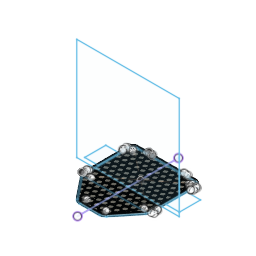
621 Chassis (Autodesk Fusion 360 design; units mm, degrees)
part number: 2026-02-18-00-04-41-213
Autodesk Fusion 360 part; units mm, degrees
note: some values were not read from the file. Set by a fixed rule: which sketch regions a step uses.
(part 1 of 3)
sketch "Sketch1" plane through (0, 0, 0) normal (0, 0, 1) x (1, 0, 0)
  line L0 (101.6, -101.6) -> (-101.6, -101.6)
  line L1 (-101.6, -101.6) -> (-101.6, 101.6)
  line L2 (-101.6, 101.6) -> (101.6, 101.6)
  line L3 (101.6, 101.6) -> (101.6, -101.6)
  line L4 (101.6, -101.6) -> (-101.6, 101.6) construction
  line L5 (-101.6, -101.6) -> (101.6, 101.6) construction
  dimension "d1" = 203.2
  dimension "d2" = 203.2
  constraint horizontal L0
  constraint perpendicular L0 L1
  constraint parallel L0 L2
  constraint parallel L1 L3
  constraint coincident L4 origin
  constraint coincident L5 origin
  measures "d1" distance of L1.end L2.end
  measures "d2" distance of L0.end L1.end
sketch "Sketch2" plane through (0, 0, 0) normal (0, 0, 1) x (1, 0, 0)
sketch "Sketch3" plane through (0, 0, 0) normal (0, 0, 1) x (1, 0, 0)
  line L0 (101.6, 101.6) -> (-101.6, 101.6)
  line L1 (-101.6, 101.6) -> (-101.6, -101.6)
  line L2 (-101.6, -101.6) -> (101.6, -101.6)
  line L3 (101.6, -101.6) -> (101.6, 101.6)
  line L4 (101.6, 101.6) -> (-101.6, -101.6) construction
  line L5 (-101.6, 101.6) -> (101.6, -101.6) construction
  dimension "d5" = 203.2
  dimension "d6" = 203.2
  constraint horizontal L0
  constraint perpendicular L0 L1
  constraint parallel L0 L2
  constraint parallel L1 L3
  constraint coincident L4 origin
  constraint coincident L5 origin
  measures "d5" distance of L1.end L2.end
  measures "d6" distance of L0.end L1.end
sketch "Sketch4" plane through (0, 0, 0) normal (0, 1, 0) x (1, 0, 0)
  line L0 (-101.6, 0) -> (101.6, 0)
  line L1 (101.6, 0) -> (101.6, -203.2)
  line L2 (101.6, -203.2) -> (-101.6, -203.2)
  line L3 (-101.6, -203.2) -> (-101.6, 0)
  dimension "d7" = 203.2
  dimension "d8" = 203.2
  constraint horizontal L0
  constraint vertical L1
  constraint horizontal L2
  constraint vertical L3
  measures "d7" distance of L0.start L0.end
  measures "d8" distance of L0.start L2.end
sketch "Sketch5" plane through (0, 0, 0) normal (0, 0, 1) x (1, 0, 0)
  line L0 (55, 75) -> (-55, 75)
  line L1 (-65, 65) -> (-65, -20.4398)
  line L2 (-65, -25) -> (65, -25)
  line L3 (65, -20.4398) -> (65, 65)
  line L4 (65, 75) -> (-65, -25) construction
  line L5 (-65, 75) -> (65, -25) construction
  line L6 (-62.1513, -28.5609) -> (-28.9032, -70.121)
  line L7 (-18.7519, -75) -> (18.7519, -75)
  line L8 (28.9032, -70.121) -> (62.1513, -28.5609)
  line L9 (67, -21.1414) -> (67, 69)
  line L10 (59, 77) -> (41, 77)
  line L11 (-67, 69) -> (-67, -9)
  line L12 (-64.1513, -29.2624) -> (-29.8644, -72.121)
  line L13 (-19.7131, -77) -> (19.7131, -77)
  line L14 (29.8644, -72.121) -> (64.1513, -29.2624)
  line L15 (-59, 77) -> (-41, 77)
  line L16 (0, 100) -> (0, -100)
  line L17 (-40, 77) -> (29, 77)
  line L18 (-30, 78) -> (-30, 81)
  line L19 (-31, 82) -> (-39, 82)
  line L20 (-40, 81) -> (-40, 78)
  line L21 (31, 82) -> (39, 82)
  line L22 (30, 78) -> (30, 81)
  line L23 (40, 81) -> (40, 78)
  arc A0 (-39, 82) -> (-40, 81) centre (-39, 81) ccw
  arc A1 (-30, 81) -> (-31, 82) centre (-31, 81) ccw
  arc A2 (-30, 78) -> (-29, 77) centre (-29, 78) ccw
  arc A3 (-41, 77) -> (-40, 78) centre (-41, 78) ccw
  arc A4 (40, 78) -> (41, 77) centre (41, 78) ccw
  arc A5 (29, 77) -> (30, 78) centre (29, 78) ccw
  line L24 (29, 77) -> (51.3644, 77)
  line L25 (-41, 77) -> (-29, 77)
  arc A6 (31, 82) -> (30, 81) centre (31, 81) ccw
  arc A7 (40, 81) -> (39, 82) centre (39, 81) ccw
  circle A8 centre (-37.5, 79.5) radius 1.5
  circle A9 centre (-32.5, 79.5) radius 1.5
  circle A10 centre (37.5, 79.5) radius 1.5
  circle A11 centre (32.5, 79.5) radius 1.5
  arc A12 (-55, 75) -> (-65, 65) centre (-55, 65) ccw
  arc A13 (-59, 77) -> (-67, 69) centre (-59, 69) ccw
  arc A14 (65, 65) -> (55, 75) centre (55, 65) ccw
  arc A15 (67, 69) -> (59, 77) centre (59, 69) ccw
  arc A16 (-29.8644, -72.121) -> (-19.7131, -77) centre (-19.7131, -64) ccw
  arc A17 (19.7131, -77) -> (29.8644, -72.121) centre (19.7131, -64) ccw
  arc A18 (18.7519, -75) -> (28.9032, -70.121) centre (18.7519, -62) ccw
  arc A19 (-28.9032, -70.121) -> (-18.7519, -75) centre (-18.7519, -62) ccw
  arc A20 (-67, -21.1414) -> (-64.1513, -29.2624) centre (-54, -21.1414) ccw
  arc A21 (-65, -20.4398) -> (-62.1513, -28.5609) centre (-52, -20.4398) ccw
  arc A22 (62.1513, -28.5609) -> (65, -20.4398) centre (52, -20.4398) ccw
  arc A23 (64.1513, -29.2624) -> (67, -21.1414) centre (54, -21.1414) ccw
  line L26 (-67.9937, -20) -> (-71, -20)
  line L27 (-72, -19) -> (-72, -11)
  line L28 (-71, -10) -> (-68, -10)
  line L29 (-67, -10) -> (-67, -20)
  circle A24 centre (-69.5, -17.5) radius 1.5
  circle A25 centre (-69.5, -12.5) radius 1.5
  arc A26 (-71, -10) -> (-72, -11) centre (-71, -11) ccw
  arc A27 (-72, -19) -> (-71, -20) centre (-71, -19) ccw
  line L30 (-66.9937, -20.9996) -> (-66.9935, -21.5528)
  arc A28 (-68, -10) -> (-67, -9) centre (-68, -9) ccw
  arc A29 (-66.9937, -20.9996) -> (-67.9937, -20) centre (-67.9937, -21) ccw
  arc A30 (72, -11) -> (71, -10) centre (71, -11) ccw
  arc A31 (71, -20) -> (72, -19) centre (71, -19) ccw
  circle A32 centre (69.5, -17.5) radius 1.5
  line L31 (67.9937, -20) -> (71, -20)
  line L32 (71, -10) -> (68, -10)
  line L33 (72, -19) -> (72, -11)
  circle A33 centre (69.5, -12.5) radius 1.5
  arc A34 (67, -9) -> (68, -10) centre (68, -9) ccw
  arc A35 (67.9937, -20) -> (66.9937, -20.9996) centre (67.9937, -21) ccw
  line L34 (-67, -9) -> (-67, -20.888)
  circle A36 centre (-69.5, -12.5) radius 1.5
  arc A37 (-72, -19) -> (-71, -20) centre (-71, -19) ccw
  line L35 (-71, -10) -> (-68, -10)
  line L36 (-72, -19) -> (-72, -11)
  circle A38 centre (-69.5, -17.5) radius 1.5
  line L37 (-67.9937, -20) -> (-71, -20)
  arc A39 (-71, -10) -> (-72, -11) centre (-71, -11) ccw
  arc A40 (-66.9937, 57.0004) -> (-67.9937, 58) centre (-67.9937, 57) ccw
  line L38 (-67.9937, 58) -> (-71, 58)
  arc A41 (-72, 59) -> (-71, 58) centre (-71, 59) ccw
  line L39 (-72, 59) -> (-72, 67)
  arc A42 (-71, 68) -> (-72, 67) centre (-71, 67) ccw
  line L40 (-71, 68) -> (-68, 68)
  arc A43 (-68, 68) -> (-67, 69) centre (-68, 69) ccw
  circle A44 centre (-69.5, 65.5) radius 1.5
  circle A45 centre (-69.5, 60.5) radius 1.5
  line L41 (-67, 68) -> (-67, 58)
  line L42 (-67, 69) -> (-67, 57.112)
  line L43 (72, 59) -> (72, 67)
  circle A46 centre (69.5, 65.5) radius 1.5
  arc A47 (67.9937, 58) -> (66.9937, 57.0004) centre (67.9937, 57) ccw
  line L44 (67, 69) -> (67, 57.112)
  line L45 (67.9937, 58) -> (71, 58)
  arc A48 (71, 58) -> (72, 59) centre (71, 59) ccw
  line L46 (71, 68) -> (68, 68)
  circle A49 centre (69.5, 60.5) radius 1.5
  arc A50 (67, 69) -> (68, 68) centre (68, 69) ccw
  line L47 (67, 68) -> (67, 58)
  arc A51 (72, 67) -> (71, 68) centre (71, 67) ccw
  point P0 (0, 25)
  point P1 (-30, 77)
  point P2 (-40, 82)
  point P3 (-72, -20)
  point P4 (72, -20)
  point P5 (-68, -9)
  point P6 (-72, -20)
  point P7 (-67.9937, -21)
  dimension "d9" = 130
  dimension "d10" = 100
  dimension "d12" = 10
  dimension "d13" = 5
  dimension "d14" = 1
  dimension "d15" = 1
  dimension "d16" = 1
  dimension "d17" = 1
  dimension "d18" = 1
  dimension "d19" = 3
  dimension "d20" = 3
  dimension "d23" = 10
  dimension "d24" = 8
  dimension "d25" = 10
  dimension "d26" = 8
  dimension "d27" = 13
  dimension "d32" = 2.5
  dimension "d33" = 2.5
  dimension "d34" = 5
  dimension "d35" = 30
  dimension "d36" = 30
  dimension "d48" = 5
  dimension "d49" = 10
  dimension "d50" = 3
  dimension "d51" = 3
  dimension "d52" = 2.5
  dimension "d53" = 5
  dimension "d54" = 2.5
  dimension "d55" = 1
  dimension "d56" = 1
  dimension "d59" = 3
  dimension "d60" = 3
  dimension "d61" = 2.5
  dimension "d62" = 5
  dimension "d63" = 2.5
  dimension "d64" = 1
  dimension "d65" = 10
  dimension "d66" = 3
  dimension "d67" = 3
  dimension "d68" = 2.5
  dimension "d69" = 5
  dimension "d70" = 2.5
  dimension "d71" = 1
  dimension "d72" = 1
  constraint horizontal L0
  constraint perpendicular L0 L1
  constraint parallel L0 L2
  constraint parallel L1 L3
  constraint coincident L4 P0
  constraint coincident L5 P0
  constraint parallel L2 L7
  constraint vertical L16
  constraint horizontal L17
  constraint vertical L18
  constraint horizontal L19
  constraint vertical L20
  constraint coincident L10 L17.start
  constraint coincident P2 L19
  constraint coincident P2 L20
  constraint tangent L19 A0
  constraint tangent L20 A0
  constraint tangent L18 A1
  constraint tangent L19 A1
  constraint equal A0 A1
  constraint coincident P1 L18
  constraint tangent L10 A2
  constraint tangent L18 A2
  constraint coincident L17.start L20
  constraint tangent L15 A3
  constraint tangent L20 A3
  constraint coincident L10 A2.end
  constraint tangent L10 A4
  constraint tangent L23 A4
  constraint coincident P1 L17
  constraint tangent L22 A5
  constraint tangent L17 A5
  constraint equal A4 A5
  constraint coincident L10 L24.end
  constraint tangent A2 L25
  constraint tangent L21 A6
  constraint tangent L22 A6
  constraint tangent L21 A7
  constraint tangent L23 A7
  constraint equal A6 A7
  constraint symmetric L16 A8 A10
  constraint symmetric L16 A9 A11
  constraint coincident L5.start L0
  constraint coincident L5.start L1
  constraint tangent L0 A12
  constraint tangent L1 A12
  constraint tangent L11 A13
  constraint tangent L15 A13
  constraint coincident L4.start L0
  constraint coincident L4.start L3
  constraint tangent L0 A14
  constraint tangent L3 A14
  constraint tangent L9 A15
  constraint tangent L10 A15
  constraint tangent L12 A16
  constraint tangent L13 A16
  constraint tangent L13 A17
  constraint tangent L14 A17
  constraint equal A16 A17
  constraint tangent L7 A18
  constraint tangent L8 A18
  constraint equal A16 A18
  constraint tangent L6 A19
  constraint tangent L7 A19
  constraint equal A16 A19
  constraint tangent L11 A20
  constraint tangent L12 A20
  constraint equal A16 A20
  constraint coincident L2.start L1
  constraint coincident L2.start L6
  constraint tangent L1 A21
  constraint tangent L6 A21
  constraint equal A16 A21
  constraint coincident L2.end L3
  constraint coincident L2.end L8
  constraint tangent L3 A22
  constraint tangent L8 A22
  constraint equal A16 A22
  constraint tangent L9 A23
  constraint tangent L14 A23
  constraint equal A16 A23
  constraint horizontal L26
  constraint vertical L27
  constraint horizontal L28
  constraint vertical L29
  constraint tangent L27 A26
  constraint tangent L28 A26
  constraint coincident P6 L26
  constraint coincident P6 L27
  constraint tangent L26 A27
  constraint tangent L27 A27
  constraint equal A26 A27
  constraint coincident A20 L30.end
  constraint coincident L11 A20.start
  constraint tangent L28 A28
  constraint tangent L11 A28
  constraint coincident L29.end L26
  constraint tangent L26 A29
  constraint tangent L30 A29
  constraint equal A28 A29
  constraint symmetric L16 P6 P4
  constraint symmetric L16 A24 A32
  constraint symmetric L16 A25 A33
  constraint symmetric L16 L27.end A30.start
  constraint symmetric L16 L28.start A30.end
  constraint symmetric L16 A26 A30
  constraint symmetric L16 L26.end A31.start
  constraint symmetric L16 L27.start A31.end
  constraint symmetric L16 A27 A31
  constraint symmetric L16 L28.end L32.end
  constraint symmetric L16 L11.end A34.start
  constraint symmetric L16 A28 A34
  constraint symmetric L16 L26.start L31.start
  constraint symmetric L16 L30.start A35.end
  constraint symmetric L16 A29 A35
  constraint coincident A29 L34.end
  constraint tangent A28 L34
  constraint horizontal L37
  constraint vertical L36
  constraint horizontal L35
  constraint tangent L36 A39
  constraint tangent L35 A39
  constraint coincident P6 L37
  constraint coincident P6 L36
  constraint tangent A37 L37
  constraint tangent A37 L36
  constraint equal A37 A39
  constraint horizontal L38
  constraint vertical L39
  constraint horizontal L40
  constraint vertical L41
  constraint tangent L39 A42
  constraint tangent A42 L40
  constraint tangent L38 A41
  constraint tangent A41 L39
  constraint equal A41 A42
  constraint tangent L40 A43
  constraint coincident L41.end L38
  constraint tangent A40 L38
  constraint equal A40 A43
  constraint coincident L42.end A40
  constraint tangent A43 L42
  constraint symmetric L16 A41.start L43.start
  constraint symmetric L16 L40.end L46.end
  constraint symmetric L16 L11.start L9.end
  constraint symmetric L16 L38.end L45.end
  constraint symmetric L16 L41.start L47.start
  constraint symmetric L16 L39.end L43.end
  constraint symmetric L16 L41.end L47.end
  constraint symmetric L16 A42.start L46.start
  constraint symmetric L16 A40.end A47.start
  constraint symmetric L16 A40.start A47.end
  constraint symmetric L16 L42.end L44.end
  constraint symmetric L16 A40 A47
  constraint symmetric L16 A41 A48
  constraint symmetric L16 A42 A51
  constraint symmetric L16 A43 A50
  constraint symmetric L16 A44 A46
  constraint symmetric L16 A45 A49
  measures "d9" distance of L2.start L2.end
  measures "d10" distance of L5.start L2.start
  measures "d12" distance of L17.start P1
  measures "d13" distance of L17.start P2
  measures "d14" radius of A0
  measures "d15" radius of A2
  measures "d16" radius of A3
  measures "d17" radius of A4
  measures "d18" radius of A6
  measures "d19" diameter of A8
  measures "d20" diameter of A9
  measures "d23" radius of A12
  measures "d24" radius of A13
  measures "d25" radius of A14
  measures "d26" radius of A15
  measures "d27" radius of A16
  measures "d32" distance of L20 A8.centre
  measures "d33" distance of L18 A9.centre
  measures "d34" distance of A8.centre A9.centre
  measures "d35" distance of L16 L22
  measures "d36" distance of L16 L18
  measures "d48" distance of L29.end P6
  measures "d49" distance of L29.end L29.start
  measures "d50" diameter of A24
  measures "d51" diameter of A25
  measures "d52" distance of L26 A24.centre
  measures "d53" distance of A24.centre A25.centre
  measures "d54" distance of L28 A25.centre
  measures "d55" radius of A26
  measures "d56" radius of A28
  measures "d59" diameter of A38
  measures "d60" diameter of A36
  measures "d61" distance of A24.centre L37
  measures "d62" distance of A25.centre A24.centre
  measures "d63" distance of A25.centre L35
  measures "d64" radius of A39
  measures "d65" distance of L41.start L41.end
  measures "d66" diameter of A45
  measures "d67" diameter of A44
  measures "d68" distance of A45.centre L38
  measures "d69" distance of A44.centre A45.centre
  measures "d70" distance of A44.centre L40
  measures "d71" radius of A42
  measures "d72" radius of A43
sketch "Wheels" plane through (0, 0, 0) normal (0, 0, 1) x (1, 0, 0)
  line L0 (-67, 50) -> (-94, 50)
  line L1 (-94, 50) -> (-94, 8)
  line L2 (-94, 8) -> (-67, 8)
  line L3 (-67, 8) -> (-67, 50)
  line L4 (0, 100) -> (0, -100)
  line L5 (94, 50) -> (94, 8)
  line L6 (67, 50) -> (94, 50)
  line L7 (94, 8) -> (67, 8)
  line L8 (67, 8) -> (67, 50)
  dimension "d21" = 27
  dimension "d22" = 42
  constraint horizontal L0
  constraint vertical L1
  constraint horizontal L2
  constraint vertical L3
  constraint symmetric L0.start L4 L6.start
  constraint symmetric L0.end L4 L5.start
  constraint symmetric L1.end L4 L5.end
  constraint symmetric L2.end L4 L7.end
  measures "d21" distance of L0.start L0.end
  measures "d22" distance of L0.start L2.end
extrude "Extrude2" add sketch "Sketch5" along normal blind 2 contours L0 L3 L7 L8 L9 L10 L13 L14 L16 L17 L24 A14 A15 A17 A18 A22 A23 L44 L47 | L0 L1 L6 L7 L11 L12 L13 L15 L16 L17 L25 A12 A13 A16 A19 A20 A21 L29 L30 A29 L34 L41 L42 makes body 1
extrude "Extrude3" add sketch "Sketch5" along normal blind 1.5 contours L17 L18 L19 L20 A0 A1 A2 A3 L25 | L21 L22 L23 A4 A5 L24 A6 A7 bodies 1
extrude "Extrude4" add 1 faces at (13.6667, 75.6667, 2) along direction (0, 0, 1) blind 2 on bodies 1 bodies 1
sketch "hex" plane through (0, 0, 0) normal (0, 0, 1) x (1, 0, 0)
  arc A0 (-55, 75) -> (-65, 65) centre (-55, 65) ccw
  line L0 (-65, 65) -> (-65, -20.4398)
  arc A1 (-65, -20.4398) -> (-62.1513, -28.5609) centre (-52, -20.4398) ccw
  line L1 (-62.1513, -28.5609) -> (-28.9032, -70.121)
  arc A2 (-28.9032, -70.121) -> (-18.7519, -75) centre (-18.7519, -62) ccw
  line L2 (-18.7519, -75) -> (18.7519, -75)
  arc A3 (18.7519, -75) -> (28.9032, -70.121) centre (18.7519, -62) ccw
  line L3 (28.9032, -70.121) -> (62.1513, -28.5609)
  arc A4 (62.1513, -28.5609) -> (65, -20.4398) centre (52, -20.4398) ccw
  line L4 (65, -20.4398) -> (65, 65)
  arc A5 (65, 65) -> (55, 75) centre (55, 65) ccw
  line L5 (55, 75) -> (-55, 75)
  line L6 (5, 2.8868) -> (0, 5.7735)
  line L7 (0, 5.7735) -> (-5, 2.8868)
  line L8 (-5, 2.8868) -> (-5, -2.8868)
  line L9 (-5, -2.8868) -> (0, -5.7735)
  line L10 (0, -5.7735) -> (5, -2.8868)
  line L11 (5, -2.8868) -> (5, 2.8868)
  line L12 (0, 0) -> (5, 0)
  line L13 (0, 0) -> (2.5, 4.3301)
  line L14 (-150, -66.9726) -> (-155, -69.8594)
  line L15 (-145, -69.8594) -> (-150, -66.9726)
  line L16 (-145, -75.6329) -> (-145, -69.8594)
  line L17 (-155, -69.8594) -> (-155, -75.6329)
  line L18 (-155, -75.6329) -> (-150, -78.5196)
  line L19 (-150, -78.5196) -> (-145, -75.6329)
  line L20 (-138, -66.9726) -> (-143, -69.8594)
  line L21 (-133, -69.8594) -> (-138, -66.9726)
  line L22 (-133, -75.6329) -> (-133, -69.8594)
  line L23 (-143, -69.8594) -> (-143, -75.6329)
  line L24 (-143, -75.6329) -> (-138, -78.5196)
  line L25 (-138, -78.5196) -> (-133, -75.6329)
  line L26 (-126, -66.9726) -> (-131, -69.8594)
  line L27 (-121, -69.8594) -> (-126, -66.9726)
  line L28 (-121, -75.6329) -> (-121, -69.8594)
  line L29 (-131, -69.8594) -> (-131, -75.6329)
  line L30 (-131, -75.6329) -> (-126, -78.5196)
  line L31 (-126, -78.5196) -> (-121, -75.6329)
  line L32 (-114, -66.9726) -> (-119, -69.8594)
  line L33 (-109, -69.8594) -> (-114, -66.9726)
  line L34 (-109, -75.6329) -> (-109, -69.8594)
  line L35 (-119, -69.8594) -> (-119, -75.6329)
  line L36 (-119, -75.6329) -> (-114, -78.5196)
  line L37 (-114, -78.5196) -> (-109, -75.6329)
  line L38 (-102, -66.9726) -> (-107, -69.8594)
  line L39 (-97, -69.8594) -> (-102, -66.9726)
  line L40 (-97, -75.6329) -> (-97, -69.8594)
  line L41 (-107, -69.8594) -> (-107, -75.6329)
  line L42 (-107, -75.6329) -> (-102, -78.5196)
  line L43 (-102, -78.5196) -> (-97, -75.6329)
  line L44 (-90, -66.9726) -> (-95, -69.8594)
  line L45 (-85, -69.8594) -> (-90, -66.9726)
  line L46 (-85, -75.6329) -> (-85, -69.8594)
  line L47 (-95, -69.8594) -> (-95, -75.6329)
  line L48 (-95, -75.6329) -> (-90, -78.5196)
  line L49 (-90, -78.5196) -> (-85, -75.6329)
  line L50 (-78, -66.9726) -> (-83, -69.8594)
  line L51 (-73, -69.8594) -> (-78, -66.9726)
  line L52 (-73, -75.6329) -> (-73, -69.8594)
  line L53 (-83, -69.8594) -> (-83, -75.6329)
  line L54 (-83, -75.6329) -> (-78, -78.5196)
  line L55 (-78, -78.5196) -> (-73, -75.6329)
  line L56 (-66, -66.9726) -> (-71, -69.8594)
  line L57 (-61, -69.8594) -> (-66, -66.9726)
  line L58 (-61, -75.6329) -> (-61, -69.8594)
  line L59 (-71, -69.8594) -> (-71, -75.6329)
  line L60 (-71, -75.6329) -> (-66, -78.5196)
  line L61 (-66, -78.5196) -> (-61, -75.6329)
  line L62 (-54, -66.9726) -> (-59, -69.8594)
  line L63 (-49, -69.8594) -> (-54, -66.9726)
  line L64 (-49, -75.6329) -> (-49, -69.8594)
  line L65 (-59, -69.8594) -> (-59, -75.6329)
  line L66 (-59, -75.6329) -> (-54, -78.5196)
  line L67 (-54, -78.5196) -> (-49, -75.6329)
  line L68 (-42, -66.9726) -> (-47, -69.8594)
  line L69 (-37, -69.8594) -> (-42, -66.9726)
  line L70 (-37, -75.6329) -> (-37, -69.8594)
  line L71 (-47, -69.8594) -> (-47, -75.6329)
  line L72 (-47, -75.6329) -> (-42, -78.5196)
  line L73 (-42, -78.5196) -> (-37, -75.6329)
  line L74 (-30, -66.9726) -> (-35, -69.8594)
  line L75 (-25, -69.8594) -> (-30, -66.9726)
  line L76 (-25, -75.6329) -> (-25, -69.8594)
  line L77 (-35, -69.8594) -> (-35, -75.6329)
  line L78 (-35, -75.6329) -> (-30, -78.5196)
  line L79 (-30, -78.5196) -> (-25, -75.6329)
  line L80 (-18, -66.9726) -> (-23, -69.8594)
  line L81 (-13, -69.8594) -> (-18, -66.9726)
  line L82 (-13, -75.6329) -> (-13, -69.8594)
  line L83 (-23, -69.8594) -> (-23, -75.6329)
  line L84 (-23, -75.6329) -> (-18, -78.5196)
  line L85 (-18, -78.5196) -> (-13, -75.6329)
  line L86 (-6, -66.9726) -> (-11, -69.8594)
  line L87 (-1, -69.8594) -> (-6, -66.9726)
  line L88 (-1, -75.6329) -> (-1, -69.8594)
  line L89 (-11, -69.8594) -> (-11, -75.6329)
  line L90 (-11, -75.6329) -> (-6, -78.5196)
  line L91 (-6, -78.5196) -> (-1, -75.6329)
  line L92 (6, -66.9726) -> (1, -69.8594)
  line L93 (11, -69.8594) -> (6, -66.9726)
  line L94 (11, -75.6329) -> (11, -69.8594)
  line L95 (1, -69.8594) -> (1, -75.6329)
  line L96 (1, -75.6329) -> (6, -78.5196)
  line L97 (6, -78.5196) -> (11, -75.6329)
  line L98 (18, -66.9726) -> (13, -69.8594)
  line L99 (23, -69.8594) -> (18, -66.9726)
  line L100 (23, -75.6329) -> (23, -69.8594)
  line L101 (13, -69.8594) -> (13, -75.6329)
  line L102 (13, -75.6329) -> (18, -78.5196)
  line L103 (18, -78.5196) -> (23, -75.6329)
  line L104 (30, -66.9726) -> (25, -69.8594)
  line L105 (35, -69.8594) -> (30, -66.9726)
  line L106 (35, -75.6329) -> (35, -69.8594)
  line L107 (25, -69.8594) -> (25, -75.6329)
  line L108 (25, -75.6329) -> (30, -78.5196)
  line L109 (30, -78.5196) -> (35, -75.6329)
  line L110 (42, -66.9726) -> (37, -69.8594)
  line L111 (47, -69.8594) -> (42, -66.9726)
  line L112 (47, -75.6329) -> (47, -69.8594)
  line L113 (37, -69.8594) -> (37, -75.6329)
  line L114 (37, -75.6329) -> (42, -78.5196)
  line L115 (42, -78.5196) -> (47, -75.6329)
  line L116 (54, -66.9726) -> (49, -69.8594)
  line L117 (59, -69.8594) -> (54, -66.9726)
  line L118 (59, -75.6329) -> (59, -69.8594)
  line L119 (49, -69.8594) -> (49, -75.6329)
  line L120 (49, -75.6329) -> (54, -78.5196)
  line L121 (54, -78.5196) -> (59, -75.6329)
  line L122 (66, -66.9726) -> (61, -69.8594)
  line L123 (71, -69.8594) -> (66, -66.9726)
  line L124 (71, -75.6329) -> (71, -69.8594)
  line L125 (61, -69.8594) -> (61, -75.6329)
  line L126 (61, -75.6329) -> (66, -78.5196)
  line L127 (66, -78.5196) -> (71, -75.6329)
  line L128 (-144, -56.5803) -> (-149, -59.4671)
  line L129 (-139, -59.4671) -> (-144, -56.5803)
  line L130 (-139, -65.2406) -> (-139, -59.4671)
  line L131 (-149, -59.4671) -> (-149, -65.2406)
  line L132 (-149, -65.2406) -> (-144, -68.1273)
  line L133 (-144, -68.1273) -> (-139, -65.2406)
  line L134 (-132, -56.5803) -> (-137, -59.4671)
  line L135 (-127, -59.4671) -> (-132, -56.5803)
  line L136 (-127, -65.2406) -> (-127, -59.4671)
  line L137 (-137, -59.4671) -> (-137, -65.2406)
  line L138 (-137, -65.2406) -> (-132, -68.1273)
  line L139 (-132, -68.1273) -> (-127, -65.2406)
  line L140 (-120, -56.5803) -> (-125, -59.4671)
  line L141 (-115, -59.4671) -> (-120, -56.5803)
  line L142 (-115, -65.2406) -> (-115, -59.4671)
  line L143 (-125, -59.4671) -> (-125, -65.2406)
  line L144 (-125, -65.2406) -> (-120, -68.1273)
  line L145 (-120, -68.1273) -> (-115, -65.2406)
  line L146 (-108, -56.5803) -> (-113, -59.4671)
  line L147 (-103, -59.4671) -> (-108, -56.5803)
  line L148 (-103, -65.2406) -> (-103, -59.4671)
  line L149 (-113, -59.4671) -> (-113, -65.2406)
  line L150 (-113, -65.2406) -> (-108, -68.1273)
  line L151 (-108, -68.1273) -> (-103, -65.2406)
  line L152 (-96, -56.5803) -> (-101, -59.4671)
  line L153 (-91, -59.4671) -> (-96, -56.5803)
  line L154 (-91, -65.2406) -> (-91, -59.4671)
  line L155 (-101, -59.4671) -> (-101, -65.2406)
  line L156 (-101, -65.2406) -> (-96, -68.1273)
  line L157 (-96, -68.1273) -> (-91, -65.2406)
  line L158 (-84, -56.5803) -> (-89, -59.4671)
  line L159 (-79, -59.4671) -> (-84, -56.5803)
  line L160 (-79, -65.2406) -> (-79, -59.4671)
  line L161 (-89, -59.4671) -> (-89, -65.2406)
  line L162 (-89, -65.2406) -> (-84, -68.1273)
  line L163 (-84, -68.1273) -> (-79, -65.2406)
  line L164 (-72, -56.5803) -> (-77, -59.4671)
  line L165 (-67, -59.4671) -> (-72, -56.5803)
  line L166 (-67, -65.2406) -> (-67, -59.4671)
  line L167 (-77, -59.4671) -> (-77, -65.2406)
  line L168 (-77, -65.2406) -> (-72, -68.1273)
  line L169 (-72, -68.1273) -> (-67, -65.2406)
  line L170 (-60, -56.5803) -> (-65, -59.4671)
  line L171 (-55, -59.4671) -> (-60, -56.5803)
  line L172 (-55, -65.2406) -> (-55, -59.4671)
  line L173 (-65, -59.4671) -> (-65, -65.2406)
  line L174 (-65, -65.2406) -> (-60, -68.1273)
  line L175 (-60, -68.1273) -> (-55, -65.2406)
  line L176 (-48, -56.5803) -> (-53, -59.4671)
  line L177 (-43, -59.4671) -> (-48, -56.5803)
  line L178 (-43, -65.2406) -> (-43, -59.4671)
  line L179 (-53, -59.4671) -> (-53, -65.2406)
  line L180 (-53, -65.2406) -> (-48, -68.1273)
  line L181 (-48, -68.1273) -> (-43, -65.2406)
  line L182 (-36, -56.5803) -> (-41, -59.4671)
  line L183 (-31, -59.4671) -> (-36, -56.5803)
  line L184 (-31, -65.2406) -> (-31, -59.4671)
  line L185 (-41, -59.4671) -> (-41, -65.2406)
  line L186 (-41, -65.2406) -> (-36, -68.1273)
  line L187 (-36, -68.1273) -> (-31, -65.2406)
  line L188 (-24, -56.5803) -> (-29, -59.4671)
  line L189 (-19, -59.4671) -> (-24, -56.5803)
  line L190 (-19, -65.2406) -> (-19, -59.4671)
  line L191 (-29, -59.4671) -> (-29, -65.2406)
  line L192 (-29, -65.2406) -> (-24, -68.1273)
  line L193 (-24, -68.1273) -> (-19, -65.2406)
  line L194 (-12, -56.5803) -> (-17, -59.4671)
  line L195 (-7, -59.4671) -> (-12, -56.5803)
  line L196 (-7, -65.2406) -> (-7, -59.4671)
  line L197 (-17, -59.4671) -> (-17, -65.2406)
  line L198 (-17, -65.2406) -> (-12, -68.1273)
  line L199 (-12, -68.1273) -> (-7, -65.2406)
  line L200 (0, -56.5803) -> (-5, -59.4671)
  line L201 (5, -59.4671) -> (0, -56.5803)
  line L202 (5, -65.2406) -> (5, -59.4671)
  line L203 (-5, -59.4671) -> (-5, -65.2406)
  line L204 (-5, -65.2406) -> (0, -68.1273)
  line L205 (0, -68.1273) -> (5, -65.2406)
  line L206 (12, -56.5803) -> (7, -59.4671)
  line L207 (17, -59.4671) -> (12, -56.5803)
  line L208 (17, -65.2406) -> (17, -59.4671)
  line L209 (7, -59.4671) -> (7, -65.2406)
  line L210 (7, -65.2406) -> (12, -68.1273)
  line L211 (12, -68.1273) -> (17, -65.2406)
  line L212 (24, -56.5803) -> (19, -59.4671)
  line L213 (29, -59.4671) -> (24, -56.5803)
  line L214 (29, -65.2406) -> (29, -59.4671)
  line L215 (19, -59.4671) -> (19, -65.2406)
  line L216 (19, -65.2406) -> (24, -68.1273)
  line L217 (24, -68.1273) -> (29, -65.2406)
  line L218 (36, -56.5803) -> (31, -59.4671)
  line L219 (41, -59.4671) -> (36, -56.5803)
  line L220 (41, -65.2406) -> (41, -59.4671)
  line L221 (31, -59.4671) -> (31, -65.2406)
  line L222 (31, -65.2406) -> (36, -68.1273)
  line L223 (36, -68.1273) -> (41, -65.2406)
  line L224 (48, -56.5803) -> (43, -59.4671)
  line L225 (53, -59.4671) -> (48, -56.5803)
  line L226 (53, -65.2406) -> (53, -59.4671)
  line L227 (43, -59.4671) -> (43, -65.2406)
  line L228 (43, -65.2406) -> (48, -68.1273)
  line L229 (48, -68.1273) -> (53, -65.2406)
  line L230 (60, -56.5803) -> (55, -59.4671)
  line L231 (65, -59.4671) -> (60, -56.5803)
  line L232 (65, -65.2406) -> (65, -59.4671)
  line L233 (55, -59.4671) -> (55, -65.2406)
  line L234 (55, -65.2406) -> (60, -68.1273)
  line L235 (60, -68.1273) -> (65, -65.2406)
  line L236 (72, -56.5803) -> (67, -59.4671)
  line L237 (77, -59.4671) -> (72, -56.5803)
  line L238 (77, -65.2406) -> (77, -59.4671)
  line L239 (67, -59.4671) -> (67, -65.2406)
  line L240 (67, -65.2406) -> (72, -68.1273)
  line L241 (72, -68.1273) -> (77, -65.2406)
  line L242 (-138, -46.188) -> (-143, -49.0748)
  line L243 (-133, -49.0748) -> (-138, -46.188)
  line L244 (-133, -54.8483) -> (-133, -49.0748)
  line L245 (-143, -49.0748) -> (-143, -54.8483)
  line L246 (-143, -54.8483) -> (-138, -57.735)
  line L247 (-138, -57.735) -> (-133, -54.8483)
  line L248 (-126, -46.188) -> (-131, -49.0748)
  line L249 (-121, -49.0748) -> (-126, -46.188)
  line L250 (-121, -54.8483) -> (-121, -49.0748)
  line L251 (-131, -49.0748) -> (-131, -54.8483)
  line L252 (-131, -54.8483) -> (-126, -57.735)
  line L253 (-126, -57.735) -> (-121, -54.8483)
  line L254 (-114, -46.188) -> (-119, -49.0748)
  line L255 (-109, -49.0748) -> (-114, -46.188)
  line L256 (-109, -54.8483) -> (-109, -49.0748)
  line L257 (-119, -49.0748) -> (-119, -54.8483)
  line L258 (-119, -54.8483) -> (-114, -57.735)
  line L259 (-114, -57.735) -> (-109, -54.8483)
  line L260 (-102, -46.188) -> (-107, -49.0748)
  line L261 (-97, -49.0748) -> (-102, -46.188)
  line L262 (-97, -54.8483) -> (-97, -49.0748)
  line L263 (-107, -49.0748) -> (-107, -54.8483)
  line L264 (-107, -54.8483) -> (-102, -57.735)
  line L265 (-102, -57.735) -> (-97, -54.8483)
  line L266 (-90, -46.188) -> (-95, -49.0748)
  line L267 (-85, -49.0748) -> (-90, -46.188)
  line L268 (-85, -54.8483) -> (-85, -49.0748)
  line L269 (-95, -49.0748) -> (-95, -54.8483)
  line L270 (-95, -54.8483) -> (-90, -57.735)
  line L271 (-90, -57.735) -> (-85, -54.8483)
  line L272 (-78, -46.188) -> (-83, -49.0748)
  line L273 (-73, -49.0748) -> (-78, -46.188)
  line L274 (-73, -54.8483) -> (-73, -49.0748)
  line L275 (-83, -49.0748) -> (-83, -54.8483)
  line L276 (-83, -54.8483) -> (-78, -57.735)
  line L277 (-78, -57.735) -> (-73, -54.8483)
  line L278 (-66, -46.188) -> (-71, -49.0748)
  line L279 (-61, -49.0748) -> (-66, -46.188)
  line L280 (-61, -54.8483) -> (-61, -49.0748)
  line L281 (-71, -49.0748) -> (-71, -54.8483)
  line L282 (-71, -54.8483) -> (-66, -57.735)
  line L283 (-66, -57.735) -> (-61, -54.8483)
  line L284 (-54, -46.188) -> (-59, -49.0748)
  line L285 (-49, -49.0748) -> (-54, -46.188)
  line L286 (-49, -54.8483) -> (-49, -49.0748)
  line L287 (-59, -49.0748) -> (-59, -54.8483)
  line L288 (-59, -54.8483) -> (-54, -57.735)
  line L289 (-54, -57.735) -> (-49, -54.8483)
  line L290 (-42, -46.188) -> (-47, -49.0748)
  line L291 (-37, -49.0748) -> (-42, -46.188)
  line L292 (-37, -54.8483) -> (-37, -49.0748)
  line L293 (-47, -49.0748) -> (-47, -54.8483)
  line L294 (-47, -54.8483) -> (-42, -57.735)
  line L295 (-42, -57.735) -> (-37, -54.8483)
  line L296 (-30, -46.188) -> (-35, -49.0748)
  line L297 (-25, -49.0748) -> (-30, -46.188)
  line L298 (-25, -54.8483) -> (-25, -49.0748)
  line L299 (-35, -49.0748) -> (-35, -54.8483)
  line L300 (-35, -54.8483) -> (-30, -57.735)
  line L301 (-30, -57.735) -> (-25, -54.8483)
  line L302 (-18, -46.188) -> (-23, -49.0748)
  line L303 (-13, -49.0748) -> (-18, -46.188)
  line L304 (-13, -54.8483) -> (-13, -49.0748)
  line L305 (-23, -49.0748) -> (-23, -54.8483)
  line L306 (-23, -54.8483) -> (-18, -57.735)
  line L307 (-18, -57.735) -> (-13, -54.8483)
  line L308 (-6, -46.188) -> (-11, -49.0748)
  line L309 (-1, -49.0748) -> (-6, -46.188)
  line L310 (-1, -54.8483) -> (-1, -49.0748)
  line L311 (-11, -49.0748) -> (-11, -54.8483)
  line L312 (-11, -54.8483) -> (-6, -57.735)
  line L313 (-6, -57.735) -> (-1, -54.8483)
  line L314 (6, -46.188) -> (1, -49.0748)
  line L315 (11, -49.0748) -> (6, -46.188)
  line L316 (11, -54.8483) -> (11, -49.0748)
  line L317 (1, -49.0748) -> (1, -54.8483)
  line L318 (1, -54.8483) -> (6, -57.735)
  line L319 (6, -57.735) -> (11, -54.8483)
  line L320 (18, -46.188) -> (13, -49.0748)
  line L321 (23, -49.0748) -> (18, -46.188)
  line L322 (23, -54.8483) -> (23, -49.0748)
  line L323 (13, -49.0748) -> (13, -54.8483)
  line L324 (13, -54.8483) -> (18, -57.735)
  line L325 (18, -57.735) -> (23, -54.8483)
  line L326 (30, -46.188) -> (25, -49.0748)
  line L327 (35, -49.0748) -> (30, -46.188)
  line L328 (35, -54.8483) -> (35, -49.0748)
  line L329 (25, -49.0748) -> (25, -54.8483)
  line L330 (25, -54.8483) -> (30, -57.735)
  line L331 (30, -57.735) -> (35, -54.8483)
  line L332 (42, -46.188) -> (37, -49.0748)
  line L333 (47, -49.0748) -> (42, -46.188)
  line L334 (47, -54.8483) -> (47, -49.0748)
  line L335 (37, -49.0748) -> (37, -54.8483)
  line L336 (37, -54.8483) -> (42, -57.735)
  line L337 (42, -57.735) -> (47, -54.8483)
  line L338 (54, -46.188) -> (49, -49.0748)
  line L339 (59, -49.0748) -> (54, -46.188)
  line L340 (59, -54.8483) -> (59, -49.0748)
  line L341 (49, -49.0748) -> (49, -54.8483)
  line L342 (49, -54.8483) -> (54, -57.735)
  line L343 (54, -57.735) -> (59, -54.8483)
  line L344 (66, -46.188) -> (61, -49.0748)
  line L345 (71, -49.0748) -> (66, -46.188)
  line L346 (71, -54.8483) -> (71, -49.0748)
  line L347 (61, -49.0748) -> (61, -54.8483)
  line L348 (61, -54.8483) -> (66, -57.735)
  line L349 (66, -57.735) -> (71, -54.8483)
  line L350 (78, -46.188) -> (73, -49.0748)
  line L351 (83, -49.0748) -> (78, -46.188)
  line L352 (83, -54.8483) -> (83, -49.0748)
  line L353 (73, -49.0748) -> (73, -54.8483)
  line L354 (73, -54.8483) -> (78, -57.735)
  line L355 (78, -57.735) -> (83, -54.8483)
  line L356 (-132, -35.7957) -> (-137, -38.6825)
  line L357 (-127, -38.6825) -> (-132, -35.7957)
  line L358 (-127, -44.456) -> (-127, -38.6825)
  line L359 (-137, -38.6825) -> (-137, -44.456)
  line L360 (-137, -44.456) -> (-132, -47.3427)
  line L361 (-132, -47.3427) -> (-127, -44.456)
  line L362 (-120, -35.7957) -> (-125, -38.6825)
  line L363 (-115, -38.6825) -> (-120, -35.7957)
  line L364 (-115, -44.456) -> (-115, -38.6825)
  line L365 (-125, -38.6825) -> (-125, -44.456)
  line L366 (-125, -44.456) -> (-120, -47.3427)
  line L367 (-120, -47.3427) -> (-115, -44.456)
  line L368 (-108, -35.7957) -> (-113, -38.6825)
  line L369 (-103, -38.6825) -> (-108, -35.7957)
  line L370 (-103, -44.456) -> (-103, -38.6825)
  line L371 (-113, -38.6825) -> (-113, -44.456)
  line L372 (-113, -44.456) -> (-108, -47.3427)
  line L373 (-108, -47.3427) -> (-103, -44.456)
  line L374 (-96, -35.7957) -> (-101, -38.6825)
  line L375 (-91, -38.6825) -> (-96, -35.7957)
  line L376 (-91, -44.456) -> (-91, -38.6825)
  line L377 (-101, -38.6825) -> (-101, -44.456)
  line L378 (-101, -44.456) -> (-96, -47.3427)
  line L379 (-96, -47.3427) -> (-91, -44.456)
  line L380 (-84, -35.7957) -> (-89, -38.6825)
  line L381 (-79, -38.6825) -> (-84, -35.7957)
  line L382 (-79, -44.456) -> (-79, -38.6825)
  line L383 (-89, -38.6825) -> (-89, -44.456)
  line L384 (-89, -44.456) -> (-84, -47.3427)
  line L385 (-84, -47.3427) -> (-79, -44.456)
  line L386 (-72, -35.7957) -> (-77, -38.6825)
  line L387 (-67, -38.6825) -> (-72, -35.7957)
  line L388 (-67, -44.456) -> (-67, -38.6825)
  line L389 (-77, -38.6825) -> (-77, -44.456)
  line L390 (-77, -44.456) -> (-72, -47.3427)
  line L391 (-72, -47.3427) -> (-67, -44.456)
  line L392 (-60, -35.7957) -> (-65, -38.6825)
  line L393 (-55, -38.6825) -> (-60, -35.7957)
  line L394 (-55, -44.456) -> (-55, -38.6825)
  line L395 (-65, -38.6825) -> (-65, -44.456)
  line L396 (-65, -44.456) -> (-60, -47.3427)
  line L397 (-60, -47.3427) -> (-55, -44.456)
  line L398 (-48, -35.7957) -> (-53, -38.6825)
  line L399 (-43, -38.6825) -> (-48, -35.7957)
  line L400 (-43, -44.456) -> (-43, -38.6825)
  line L401 (-53, -38.6825) -> (-53, -44.456)
  line L402 (-53, -44.456) -> (-48, -47.3427)
  line L403 (-48, -47.3427) -> (-43, -44.456)
  line L404 (-36, -35.7957) -> (-41, -38.6825)
  line L405 (-31, -38.6825) -> (-36, -35.7957)
  line L406 (-31, -44.456) -> (-31, -38.6825)
  line L407 (-41, -38.6825) -> (-41, -44.456)
  line L408 (-41, -44.456) -> (-36, -47.3427)
  line L409 (-36, -47.3427) -> (-31, -44.456)
  line L410 (-24, -35.7957) -> (-29, -38.6825)
  line L411 (-19, -38.6825) -> (-24, -35.7957)
  line L412 (-19, -44.456) -> (-19, -38.6825)
  line L413 (-29, -38.6825) -> (-29, -44.456)
  line L414 (-29, -44.456) -> (-24, -47.3427)
  line L415 (-24, -47.3427) -> (-19, -44.456)
  line L416 (-12, -35.7957) -> (-17, -38.6825)
  line L417 (-7, -38.6825) -> (-12, -35.7957)
  line L418 (-7, -44.456) -> (-7, -38.6825)
  line L419 (-17, -38.6825) -> (-17, -44.456)
  line L420 (-17, -44.456) -> (-12, -47.3427)
  line L421 (-12, -47.3427) -> (-7, -44.456)
  line L422 (0, -35.7957) -> (-5, -38.6825)
  line L423 (5, -38.6825) -> (0, -35.7957)
  line L424 (5, -44.456) -> (5, -38.6825)
  line L425 (-5, -38.6825) -> (-5, -44.456)
  line L426 (-5, -44.456) -> (0, -47.3427)
  line L427 (0, -47.3427) -> (5, -44.456)
  line L428 (12, -35.7957) -> (7, -38.6825)
  line L429 (17, -38.6825) -> (12, -35.7957)
  line L430 (17, -44.456) -> (17, -38.6825)
  line L431 (7, -38.6825) -> (7, -44.456)
  line L432 (7, -44.456) -> (12, -47.3427)
  line L433 (12, -47.3427) -> (17, -44.456)
  line L434 (24, -35.7957) -> (19, -38.6825)
  line L435 (29, -38.6825) -> (24, -35.7957)
  line L436 (29, -44.456) -> (29, -38.6825)
  line L437 (19, -38.6825) -> (19, -44.456)
  line L438 (19, -44.456) -> (24, -47.3427)
  line L439 (24, -47.3427) -> (29, -44.456)
  line L440 (36, -35.7957) -> (31, -38.6825)
  line L441 (41, -38.6825) -> (36, -35.7957)
  line L442 (41, -44.456) -> (41, -38.6825)
  line L443 (31, -38.6825) -> (31, -44.456)
  line L444 (31, -44.456) -> (36, -47.3427)
  line L445 (36, -47.3427) -> (41, -44.456)
  line L446 (48, -35.7957) -> (43, -38.6825)
  line L447 (53, -38.6825) -> (48, -35.7957)
  line L448 (53, -44.456) -> (53, -38.6825)
  line L449 (43, -38.6825) -> (43, -44.456)
  line L450 (43, -44.456) -> (48, -47.3427)
  line L451 (48, -47.3427) -> (53, -44.456)
  line L452 (60, -35.7957) -> (55, -38.6825)
  line L453 (65, -38.6825) -> (60, -35.7957)
  line L454 (65, -44.456) -> (65, -38.6825)
  line L455 (55, -38.6825) -> (55, -44.456)
  line L456 (55, -44.456) -> (60, -47.3427)
  line L457 (60, -47.3427) -> (65, -44.456)
  line L458 (72, -35.7957) -> (67, -38.6825)
  line L459 (77, -38.6825) -> (72, -35.7957)
  line L460 (77, -44.456) -> (77, -38.6825)
  line L461 (67, -38.6825) -> (67, -44.456)
  line L462 (67, -44.456) -> (72, -47.3427)
  line L463 (72, -47.3427) -> (77, -44.456)
  line L464 (84, -35.7957) -> (79, -38.6825)
  line L465 (89, -38.6825) -> (84, -35.7957)
  line L466 (89, -44.456) -> (89, -38.6825)
  line L467 (79, -38.6825) -> (79, -44.456)
  line L468 (79, -44.456) -> (84, -47.3427)
  line L469 (84, -47.3427) -> (89, -44.456)
  line L470 (-126, -25.4034) -> (-131, -28.2902)
  line L471 (-121, -28.2902) -> (-126, -25.4034)
  line L472 (-121, -34.0637) -> (-121, -28.2902)
  line L473 (-131, -28.2902) -> (-131, -34.0637)
  line L474 (-131, -34.0637) -> (-126, -36.9504)
  line L475 (-126, -36.9504) -> (-121, -34.0637)
  line L476 (-114, -25.4034) -> (-119, -28.2902)
  line L477 (-109, -28.2902) -> (-114, -25.4034)
  line L478 (-109, -34.0637) -> (-109, -28.2902)
  line L479 (-119, -28.2902) -> (-119, -34.0637)
  line L480 (-119, -34.0637) -> (-114, -36.9504)
  line L481 (-114, -36.9504) -> (-109, -34.0637)
  line L482 (-102, -25.4034) -> (-107, -28.2902)
  line L483 (-97, -28.2902) -> (-102, -25.4034)
  line L484 (-97, -34.0637) -> (-97, -28.2902)
  line L485 (-107, -28.2902) -> (-107, -34.0637)
  line L486 (-107, -34.0637) -> (-102, -36.9504)
  line L487 (-102, -36.9504) -> (-97, -34.0637)
  line L488 (-90, -25.4034) -> (-95, -28.2902)
  line L489 (-85, -28.2902) -> (-90, -25.4034)
  line L490 (-85, -34.0637) -> (-85, -28.2902)
  line L491 (-95, -28.2902) -> (-95, -34.0637)
  line L492 (-95, -34.0637) -> (-90, -36.9504)
  line L493 (-90, -36.9504) -> (-85, -34.0637)
  line L494 (-78, -25.4034) -> (-83, -28.2902)
  line L495 (-73, -28.2902) -> (-78, -25.4034)
  line L496 (-73, -34.0637) -> (-73, -28.2902)
  line L497 (-83, -28.2902) -> (-83, -34.0637)
  line L498 (-83, -34.0637) -> (-78, -36.9504)
  line L499 (-78, -36.9504) -> (-73, -34.0637)
  line L500 (-66, -25.4034) -> (-71, -28.2902)
  line L501 (-61, -28.2902) -> (-66, -25.4034)
  line L502 (-61, -34.0637) -> (-61, -28.2902)
  line L503 (-71, -28.2902) -> (-71, -34.0637)
  line L504 (-71, -34.0637) -> (-66, -36.9504)
  line L505 (-66, -36.9504) -> (-61, -34.0637)
  line L506 (-54, -25.4034) -> (-59, -28.2902)
  line L507 (-49, -28.2902) -> (-54, -25.4034)
  line L508 (-49, -34.0637) -> (-49, -28.2902)
  line L509 (-59, -28.2902) -> (-59, -34.0637)
  line L510 (-59, -34.0637) -> (-54, -36.9504)
  line L511 (-54, -36.9504) -> (-49, -34.0637)
  line L512 (-42, -25.4034) -> (-47, -28.2902)
  line L513 (-37, -28.2902) -> (-42, -25.4034)
  line L514 (-37, -34.0637) -> (-37, -28.2902)
  line L515 (-47, -28.2902) -> (-47, -34.0637)
  line L516 (-47, -34.0637) -> (-42, -36.9504)
  line L517 (-42, -36.9504) -> (-37, -34.0637)
  line L518 (-30, -25.4034) -> (-35, -28.2902)
  line L519 (-25, -28.2902) -> (-30, -25.4034)
  line L520 (-25, -34.0637) -> (-25, -28.2902)
  line L521 (-35, -28.2902) -> (-35, -34.0637)
  line L522 (-35, -34.0637) -> (-30, -36.9504)
  line L523 (-30, -36.9504) -> (-25, -34.0637)
  line L524 (-18, -25.4034) -> (-23, -28.2902)
  line L525 (-13, -28.2902) -> (-18, -25.4034)
  line L526 (-13, -34.0637) -> (-13, -28.2902)
  line L527 (-23, -28.2902) -> (-23, -34.0637)
  line L528 (-23, -34.0637) -> (-18, -36.9504)
  line L529 (-18, -36.9504) -> (-13, -34.0637)
  line L530 (-6, -25.4034) -> (-11, -28.2902)
  line L531 (-1, -28.2902) -> (-6, -25.4034)
  line L532 (-1, -34.0637) -> (-1, -28.2902)
  line L533 (-11, -28.2902) -> (-11, -34.0637)
  line L534 (-11, -34.0637) -> (-6, -36.9504)
  line L535 (-6, -36.9504) -> (-1, -34.0637)
  line L536 (6, -25.4034) -> (1, -28.2902)
  line L537 (11, -28.2902) -> (6, -25.4034)
  line L538 (11, -34.0637) -> (11, -28.2902)
  line L539 (1, -28.2902) -> (1, -34.0637)
  line L540 (1, -34.0637) -> (6, -36.9504)
  line L541 (6, -36.9504) -> (11, -34.0637)
  line L542 (18, -25.4034) -> (13, -28.2902)
  line L543 (23, -28.2902) -> (18, -25.4034)
  line L544 (23, -34.0637) -> (23, -28.2902)
  line L545 (13, -28.2902) -> (13, -34.0637)
  line L546 (13, -34.0637) -> (18, -36.9504)
  line L547 (18, -36.9504) -> (23, -34.0637)
  line L548 (30, -25.4034) -> (25, -28.2902)
  line L549 (35, -28.2902) -> (30, -25.4034)
  line L550 (35, -34.0637) -> (35, -28.2902)
  line L551 (25, -28.2902) -> (25, -34.0637)
  line L552 (25, -34.0637) -> (30, -36.9504)
  line L553 (30, -36.9504) -> (35, -34.0637)
  line L554 (42, -25.4034) -> (37, -28.2902)
  line L555 (47, -28.2902) -> (42, -25.4034)
  line L556 (47, -34.0637) -> (47, -28.2902)
  line L557 (37, -28.2902) -> (37, -34.0637)
  line L558 (37, -34.0637) -> (42, -36.9504)
  line L559 (42, -36.9504) -> (47, -34.0637)
  line L560 (54, -25.4034) -> (49, -28.2902)
  line L561 (59, -28.2902) -> (54, -25.4034)
  line L562 (59, -34.0637) -> (59, -28.2902)
  line L563 (49, -28.2902) -> (49, -34.0637)
  line L564 (49, -34.0637) -> (54, -36.9504)
  line L565 (54, -36.9504) -> (59, -34.0637)
  line L566 (66, -25.4034) -> (61, -28.2902)
  line L567 (71, -28.2902) -> (66, -25.4034)
  line L568 (71, -34.0637) -> (71, -28.2902)
  line L569 (61, -28.2902) -> (61, -34.0637)
  line L570 (61, -34.0637) -> (66, -36.9504)
  line L571 (66, -36.9504) -> (71, -34.0637)
  line L572 (78, -25.4034) -> (73, -28.2902)
  line L573 (83, -28.2902) -> (78, -25.4034)
  line L574 (83, -34.0637) -> (83, -28.2902)
  line L575 (73, -28.2902) -> (73, -34.0637)
  line L576 (73, -34.0637) -> (78, -36.9504)
  line L577 (78, -36.9504) -> (83, -34.0637)
  line L578 (90, -25.4034) -> (85, -28.2902)
  line L579 (95, -28.2902) -> (90, -25.4034)
  line L580 (95, -34.0637) -> (95, -28.2902)
  line L581 (85, -28.2902) -> (85, -34.0637)
  line L582 (85, -34.0637) -> (90, -36.9504)
  line L583 (90, -36.9504) -> (95, -34.0637)
  line L584 (-120, -15.0111) -> (-125, -17.8979)
  line L585 (-115, -17.8979) -> (-120, -15.0111)
  line L586 (-115, -23.6714) -> (-115, -17.8979)
  line L587 (-125, -17.8979) -> (-125, -23.6714)
  line L588 (-125, -23.6714) -> (-120, -26.5581)
  line L589 (-120, -26.5581) -> (-115, -23.6714)
  line L590 (-108, -15.0111) -> (-113, -17.8979)
  line L591 (-103, -17.8979) -> (-108, -15.0111)
  line L592 (-103, -23.6714) -> (-103, -17.8979)
  line L593 (-113, -17.8979) -> (-113, -23.6714)
  line L594 (-113, -23.6714) -> (-108, -26.5581)
  line L595 (-108, -26.5581) -> (-103, -23.6714)
  line L596 (-96, -15.0111) -> (-101, -17.8979)
  line L597 (-91, -17.8979) -> (-96, -15.0111)
  line L598 (-91, -23.6714) -> (-91, -17.8979)
  line L599 (-101, -17.8979) -> (-101, -23.6714)
  line L600 (-101, -23.6714) -> (-96, -26.5581)
  line L601 (-96, -26.5581) -> (-91, -23.6714)
  line L602 (-84, -15.0111) -> (-89, -17.8979)
  line L603 (-79, -17.8979) -> (-84, -15.0111)
  line L604 (-79, -23.6714) -> (-79, -17.8979)
  line L605 (-89, -17.8979) -> (-89, -23.6714)
  line L606 (-89, -23.6714) -> (-84, -26.5581)
  line L607 (-84, -26.5581) -> (-79, -23.6714)
  line L608 (-72, -15.0111) -> (-77, -17.8979)
  line L609 (-67, -17.8979) -> (-72, -15.0111)
  line L610 (-67, -23.6714) -> (-67, -17.8979)
  line L611 (-77, -17.8979) -> (-77, -23.6714)
  line L612 (-77, -23.6714) -> (-72, -26.5581)
  line L613 (-72, -26.5581) -> (-67, -23.6714)
  line L614 (-60, -15.0111) -> (-65, -17.8979)
  line L615 (-55, -17.8979) -> (-60, -15.0111)
  line L616 (-55, -23.6714) -> (-55, -17.8979)
  line L617 (-65, -17.8979) -> (-65, -23.6714)
  line L618 (-65, -23.6714) -> (-60, -26.5581)
  line L619 (-60, -26.5581) -> (-55, -23.6714)
  line L620 (-48, -15.0111) -> (-53, -17.8979)
  line L621 (-43, -17.8979) -> (-48, -15.0111)
  line L622 (-43, -23.6714) -> (-43, -17.8979)
  line L623 (-53, -17.8979) -> (-53, -23.6714)
  line L624 (-53, -23.6714) -> (-48, -26.5581)
  line L625 (-48, -26.5581) -> (-43, -23.6714)
  line L626 (-36, -15.0111) -> (-41, -17.8979)
  line L627 (-31, -17.8979) -> (-36, -15.0111)
  line L628 (-31, -23.6714) -> (-31, -17.8979)
  line L629 (-41, -17.8979) -> (-41, -23.6714)
  line L630 (-41, -23.6714) -> (-36, -26.5581)
  line L631 (-36, -26.5581) -> (-31, -23.6714)
  line L632 (-24, -15.0111) -> (-29, -17.8979)
  line L633 (-19, -17.8979) -> (-24, -15.0111)
  line L634 (-19, -23.6714) -> (-19, -17.8979)
  line L635 (-29, -17.8979) -> (-29, -23.6714)
  line L636 (-29, -23.6714) -> (-24, -26.5581)
  line L637 (-24, -26.5581) -> (-19, -23.6714)
  line L638 (-12, -15.0111) -> (-17, -17.8979)
  line L639 (-7, -17.8979) -> (-12, -15.0111)
  line L640 (-7, -23.6714) -> (-7, -17.8979)
  line L641 (-17, -17.8979) -> (-17, -23.6714)
  line L642 (-17, -23.6714) -> (-12, -26.5581)
  line L643 (-12, -26.5581) -> (-7, -23.6714)
  line L644 (0, -15.0111) -> (-5, -17.8979)
  line L645 (5, -17.8979) -> (0, -15.0111)
  line L646 (5, -23.6714) -> (5, -17.8979)
  line L647 (-5, -17.8979) -> (-5, -23.6714)
  line L648 (-5, -23.6714) -> (0, -26.5581)
  line L649 (0, -26.5581) -> (5, -23.6714)
  line L650 (12, -15.0111) -> (7, -17.8979)
  line L651 (17, -17.8979) -> (12, -15.0111)
  line L652 (17, -23.6714) -> (17, -17.8979)
  line L653 (7, -17.8979) -> (7, -23.6714)
  line L654 (7, -23.6714) -> (12, -26.5581)
  line L655 (12, -26.5581) -> (17, -23.6714)
  line L656 (24, -15.0111) -> (19, -17.8979)
  line L657 (29, -17.8979) -> (24, -15.0111)
  line L658 (29, -23.6714) -> (29, -17.8979)
  line L659 (19, -17.8979) -> (19, -23.6714)
  line L660 (19, -23.6714) -> (24, -26.5581)
  line L661 (24, -26.5581) -> (29, -23.6714)
  line L662 (36, -15.0111) -> (31, -17.8979)
  line L663 (41, -17.8979) -> (36, -15.0111)
  line L664 (41, -23.6714) -> (41, -17.8979)
  line L665 (31, -17.8979) -> (31, -23.6714)
  line L666 (31, -23.6714) -> (36, -26.5581)
  line L667 (36, -26.5581) -> (41, -23.6714)
  line L668 (48, -15.0111) -> (43, -17.8979)
  line L669 (53, -17.8979) -> (48, -15.0111)
  line L670 (53, -23.6714) -> (53, -17.8979)
  line L671 (43, -17.8979) -> (43, -23.6714)
  line L672 (43, -23.6714) -> (48, -26.5581)
  line L673 (48, -26.5581) -> (53, -23.6714)
  line L674 (60, -15.0111) -> (55, -17.8979)
  line L675 (65, -17.8979) -> (60, -15.0111)
  line L676 (65, -23.6714) -> (65, -17.8979)
  line L677 (55, -17.8979) -> (55, -23.6714)
  line L678 (55, -23.6714) -> (60, -26.5581)
  line L679 (60, -26.5581) -> (65, -23.6714)
  line L680 (72, -15.0111) -> (67, -17.8979)
  line L681 (77, -17.8979) -> (72, -15.0111)
  line L682 (77, -23.6714) -> (77, -17.8979)
  line L683 (67, -17.8979) -> (67, -23.6714)
  line L684 (67, -23.6714) -> (72, -26.5581)
  line L685 (72, -26.5581) -> (77, -23.6714)
  line L686 (84, -15.0111) -> (79, -17.8979)
  line L687 (89, -17.8979) -> (84, -15.0111)
  line L688 (89, -23.6714) -> (89, -17.8979)
  line L689 (79, -17.8979) -> (79, -23.6714)
  line L690 (79, -23.6714) -> (84, -26.5581)
  line L691 (84, -26.5581) -> (89, -23.6714)
  line L692 (96, -15.0111) -> (91, -17.8979)
  line L693 (101, -17.8979) -> (96, -15.0111)
  line L694 (101, -23.6714) -> (101, -17.8979)
  line L695 (91, -17.8979) -> (91, -23.6714)
  line L696 (91, -23.6714) -> (96, -26.5581)
  line L697 (96, -26.5581) -> (101, -23.6714)
  line L698 (-114, -4.6188) -> (-119, -7.5056)
  line L699 (-109, -7.5056) -> (-114, -4.6188)
  line L700 (-109, -13.2791) -> (-109, -7.5056)
  line L701 (-119, -7.5056) -> (-119, -13.2791)
  line L702 (-119, -13.2791) -> (-114, -16.1658)
  line L703 (-114, -16.1658) -> (-109, -13.2791)
  line L704 (-102, -4.6188) -> (-107, -7.5056)
  line L705 (-97, -7.5056) -> (-102, -4.6188)
  line L706 (-97, -13.2791) -> (-97, -7.5056)
  line L707 (-107, -7.5056) -> (-107, -13.2791)
  line L708 (-107, -13.2791) -> (-102, -16.1658)
  line L709 (-102, -16.1658) -> (-97, -13.2791)
  line L710 (-90, -4.6188) -> (-95, -7.5056)
  line L711 (-85, -7.5056) -> (-90, -4.6188)
  line L712 (-85, -13.2791) -> (-85, -7.5056)
  line L713 (-95, -7.5056) -> (-95, -13.2791)
  line L714 (-95, -13.2791) -> (-90, -16.1658)
  line L715 (-90, -16.1658) -> (-85, -13.2791)
  line L716 (-78, -4.6188) -> (-83, -7.5056)
  line L717 (-73, -7.5056) -> (-78, -4.6188)
  line L718 (-73, -13.2791) -> (-73, -7.5056)
  line L719 (-83, -7.5056) -> (-83, -13.2791)
  line L720 (-83, -13.2791) -> (-78, -16.1658)
  line L721 (-78, -16.1658) -> (-73, -13.2791)
  line L722 (-66, -4.6188) -> (-71, -7.5056)